Autodesk Fusion 360 part; units mm, degrees
(part 15 of 20)
  line L330 (29.8938, -739.4997) -> (29.2799, -739.4997)
  line L331 (20.1598, -739.4999) -> (19.5459, -739.4999)
  line L332 (19.5459, -739.4999) -> (19.5458, -735.5879)
  spline S948 degree 3 poles (19.5458, -735.5879) (19.4621, -735.6608) (19.2807, -735.8186) (19.0751, -735.9436) (18.9643, -736.0109) knots 0 0 0 0 0.033221 0.072019 0.072019 0.072019 0.072019
  spline S949 degree 3 poles (18.9643, -736.0109) (18.8518, -736.0753) (18.6431, -736.1948) (18.4206, -736.286) (18.318, -736.3281) knots 0 0 0 0 0.03884 0.072064 0.072064 0.072064 0.072064
  line L333 (18.318, -736.3281) -> (18.318, -735.7346)
  spline S950 degree 3 poles (18.318, -735.7346) (18.4826, -735.6511) (18.804, -735.488) (19.0825, -735.2595) (19.2184, -735.148) knots 0 0 0 0 0.05519 0.10775 0.10775 0.10775 0.10775
  spline S951 degree 3 poles (19.2184, -735.148) (19.3344, -735.0399) (19.5471, -734.8418) (19.6962, -734.5927) (19.7641, -734.4795) knots 0 0 0 0 0.047275 0.086674 0.086674 0.086674 0.086674
  line L334 (19.7641, -734.4795) -> (20.1597, -734.4795)
  line L335 (20.1597, -734.4795) -> (20.1598, -739.4999)
  line L336 (28.5502, -789.465) -> (28.5499, -785.8429)
  line L337 (28.5499, -785.8429) -> (29.0991, -785.8429)
  line L338 (29.0991, -785.8429) -> (29.0991, -786.3511)
  spline S952 degree 3 poles (29.0991, -786.3511) (29.161, -786.2665) (29.2859, -786.096) (29.4633, -785.981) (29.5527, -785.923) knots 0 0 0 0 0.031158 0.062835 0.062835 0.062835 0.062835
  spline S953 degree 3 poles (29.5527, -785.923) (29.6519, -785.8758) (29.8557, -785.7786) (30.0814, -785.767) (30.1973, -785.761) knots 0 0 0 0 0.032617 0.067048 0.067048 0.067048 0.067048
  spline S954 degree 3 poles (30.1973, -785.761) (30.3218, -785.7657) (30.5542, -785.7745) (30.7612, -785.8794) (30.8572, -785.928) knots 0 0 0 0 0.036859 0.068796 0.068796 0.068796 0.068796
  spline S955 degree 3 poles (30.8572, -785.928) (30.9369, -785.9898) (31.0979, -786.1144) (31.1794, -786.301) (31.2205, -786.3953) knots 0 0 0 0 0.029725 0.060035 0.060035 0.060035 0.060035
  spline S956 degree 3 poles (31.2205, -786.3953) (31.3707, -786.2103) (31.6618, -785.8517) (32.1182, -785.7905) (32.3392, -785.7608) knots 0 0 0 0 0.068625 0.133023 0.133023 0.133023 0.133023
  spline S957 degree 3 poles (32.3392, -785.7608) (32.5042, -785.7692) (32.8121, -785.7849) (33.0552, -785.9723) (33.168, -786.0592) knots 0 0 0 0 0.048244 0.08997 0.08997 0.08997 0.08997
  spline S958 degree 3 poles (33.168, -786.0592) (33.2523, -786.1815) (33.4417, -786.4564) (33.4522, -786.792) (33.4579, -786.9783) knots 0 0 0 0 0.043695 0.098195 0.098195 0.098195 0.098195
  line L339 (33.4579, -786.9783) -> (33.4581, -789.4647)
  line L340 (33.4581, -789.4647) -> (32.8476, -789.4647)
  line L341 (32.8476, -789.4647) -> (32.8475, -787.183)
  spline S959 degree 3 poles (32.8475, -787.183) (32.8474, -787.0768) (32.8474, -786.8975) (32.805, -786.7235) (32.7877, -786.6526) knots 0 0 0 0 0.031711 0.053535 0.053535 0.053535 0.053535
  spline S960 degree 3 poles (32.7877, -786.6526) (32.7633, -786.601) (32.7134, -786.4956) (32.6192, -786.4268) (32.5711, -786.3918) knots 0 0 0 0 0.016863 0.034394 0.034394 0.034394 0.034394
  spline S961 degree 3 poles (32.5711, -786.3918) (32.5154, -786.3629) (32.4, -786.3032) (32.27, -786.2964) (32.2028, -786.2929) knots 0 0 0 0 0.018597 0.038532 0.038532 0.038532 0.038532
  spline S962 degree 3 poles (32.2028, -786.2929) (32.0816, -786.3027) (31.8437, -786.3219) (31.6591, -786.4729) (31.5684, -786.547) knots 0 0 0 0 0.035532 0.069798 0.069798 0.069798 0.069798
  spline S963 degree 3 poles (31.5684, -786.547) (31.4951, -786.6537) (31.328, -786.8969) (31.3204, -787.1938) (31.3161, -787.3605) knots 0 0 0 0 0.038079 0.086792 0.086792 0.086792 0.086792
  line L342 (31.3161, -787.3605) -> (31.3162, -789.4648)
  line L343 (31.3162, -789.4648) -> (30.7023, -789.4649)
  line L344 (30.7023, -789.4649) -> (30.7022, -787.1115)
  spline S964 degree 3 poles (30.7022, -787.1115) (30.6997, -786.9895) (30.6954, -786.7727) (30.5956, -786.5813) (30.552, -786.4976) knots 0 0 0 0 0.036008 0.063954 0.063954 0.063954 0.063954
  spline S965 degree 3 poles (30.552, -786.4976) (30.4898, -786.4381) (30.3536, -786.3077) (30.1639, -786.2982) (30.0609, -786.293) knots 0 0 0 0 0.025037 0.054812 0.054812 0.054812 0.054812
  spline S966 degree 3 poles (30.0609, -786.293) (29.9761, -786.2987) (29.8067, -786.3101) (29.6567, -786.3897) (29.5817, -786.4295) knots 0 0 0 0 0.025172 0.050327 0.050327 0.050327 0.050327
  spline S967 degree 3 poles (29.5817, -786.4295) (29.5131, -786.4812) (29.3728, -786.5868) (29.3, -786.7468) (29.2628, -786.8286) knots 0 0 0 0 0.025339 0.051812 0.051812 0.051812 0.051812
  spline S968 degree 3 poles (29.2628, -786.8286) (29.2341, -786.9349) (29.1673, -787.1824) (29.1652, -787.4392) (29.164, -787.5857) knots 0 0 0 0 0.032907 0.076633 0.076633 0.076633 0.076633
  line L345 (29.164, -787.5857) -> (29.1641, -789.465)
  line L346 (29.1641, -789.465) -> (28.5502, -789.465)
  line L347 (27.416, -838.1729) -> (28.0197, -838.2513)
  spline S969 degree 3 poles (28.0197, -838.2513) (27.9771, -838.4452) (27.8953, -838.817) (27.6369, -839.0953) (27.5133, -839.2285) knots 0 0 0 0 0.058356 0.111856 0.111856 0.111856 0.111856
  spline S970 degree 3 poles (27.5133, -839.2285) (27.3672, -839.3314) (27.0671, -839.5429) (26.7004, -839.5684) (26.5123, -839.5815) knots 0 0 0 0 0.052559 0.107965 0.107965 0.107965 0.107965
  spline S971 degree 3 poles (26.5123, -839.5815) (26.2792, -839.564) (25.8276, -839.5301) (25.4834, -839.2373) (25.3168, -839.0956) knots 0 0 0 0 0.068154 0.132052 0.132052 0.132052 0.132052
  spline S972 degree 3 poles (25.3168, -839.0956) (25.1853, -838.9048) (24.8974, -838.4874) (24.8763, -837.9786) (24.8649, -837.7023) knots 0 0 0 0 0.068157 0.149141 0.149141 0.149141 0.149141
  spline S973 degree 3 poles (24.8649, -837.7023) (24.8712, -837.5171) (24.8832, -837.1646) (25.0026, -836.833) (25.0592, -836.6757) knots 0 0 0 0 0.055211 0.105055 0.105055 0.105055 0.105055
  spline S974 degree 3 poles (25.0592, -836.6757) (25.1314, -836.5388) (25.2736, -836.2692) (25.5265, -836.0993) (25.651, -836.0157) knots 0 0 0 0 0.04564 0.089884 0.089884 0.089884 0.089884
  spline S975 degree 3 poles (25.651, -836.0157) (25.7869, -835.9516) (26.0608, -835.8223) (26.3632, -835.8046) (26.5156, -835.7957) knots 0 0 0 0 0.044643 0.089955 0.089955 0.089955 0.089955
  spline S976 degree 3 poles (26.5156, -835.7957) (26.6993, -835.8051) (27.0472, -835.8228) (27.3418, -836.0071) (27.4808, -836.0941) knots 0 0 0 0 0.054149 0.102527 0.102527 0.102527 0.102527
  spline S977 degree 3 poles (27.4808, -836.0941) (27.5953, -836.2076) (27.8343, -836.4446) (27.9181, -836.7714) (27.9617, -836.9416) knots 0 0 0 0 0.047449 0.099081 0.099081 0.099081 0.099081
  line L348 (27.9617, -836.9416) -> (27.3648, -837.0337)
  spline S978 degree 3 poles (27.3648, -837.0337) (27.334, -836.9224) (27.2765, -836.7149) (27.1306, -836.5575) (27.063, -836.4846) knots 0 0 0 0 0.034086 0.063475 0.063475 0.063475 0.063475
  spline S979 degree 3 poles (27.063, -836.4846) (26.986, -836.4309) (26.8287, -836.3212) (26.6372, -836.3075) (26.5394, -836.3005) knots 0 0 0 0 0.027619 0.056426 0.056426 0.056426 0.056426
  spline S980 degree 3 poles (26.5394, -836.3005) (26.3928, -836.3135) (26.1037, -836.3393) (25.8907, -836.5361) (25.7857, -836.6331) knots 0 0 0 0 0.04285 0.084486 0.084486 0.084486 0.084486
  spline S981 degree 3 poles (25.7857, -836.6331) (25.7015, -836.7726) (25.5077, -837.0941) (25.5001, -837.4716) (25.4958, -837.6852) knots 0 0 0 0 0.048123 0.11083 0.11083 0.11083 0.11083
  spline S982 degree 3 poles (25.4958, -837.6852) (25.4994, -837.901) (25.5057, -838.2797) (25.6944, -838.6057) (25.7755, -838.7459) knots 0 0 0 0 0.063398 0.111295 0.111295 0.111295 0.111295
  spline S983 degree 3 poles (25.7755, -838.7459) (25.8767, -838.8424) (26.0813, -839.0376) (26.363, -839.0636) (26.5054, -839.0768) knots 0 0 0 0 0.040675 0.082263 0.082263 0.082263 0.082263
  spline S984 degree 3 poles (26.5054, -839.0768) (26.6198, -839.0685) (26.8427, -839.0525) (27.0219, -838.9197) (27.1091, -838.855) knots 0 0 0 0 0.033628 0.065508 0.065508 0.065508 0.065508
  spline S985 degree 3 poles (27.1091, -838.855) (27.1832, -838.7651) (27.3466, -838.5664) (27.3915, -838.312) (27.416, -838.1729) knots 0 0 0 0 0.034396 0.07593 0.07593 0.07593 0.07593
  spline S986 degree 3 poles (19.0565, -837.034) (19.0601, -836.7657) (19.0666, -836.2825) (19.1859, -835.8147) (19.2389, -835.6067) knots 0 0 0 0 0.080152 0.144341 0.144341 0.144341 0.144341
  spline S987 degree 3 poles (19.2389, -835.6067) (19.3036, -835.4398) (19.4261, -835.1233) (19.6672, -834.8853) (19.7812, -834.7728) knots 0 0 0 0 0.052977 0.10048 0.10048 0.10048 0.10048
  spline S988 degree 3 poles (19.7812, -834.7728) (19.9126, -834.6872) (20.1874, -834.5083) (20.5155, -834.4893) (20.6867, -834.4794) knots 0 0 0 0 0.046203 0.096661 0.096661 0.096661 0.096661
  spline S989 degree 3 poles (20.6867, -834.4794) (20.8145, -834.485) (21.06, -834.4957) (21.2849, -834.5942) (21.3927, -834.6414) knots 0 0 0 0 0.037989 0.072993 0.072993 0.072993 0.072993
  spline S990 degree 3 poles (21.3927, -834.6414) (21.49, -834.7021) (21.6873, -834.8253) (21.8245, -835.0133) (21.8941, -835.1086) knots 0 0 0 0 0.034048 0.069103 0.069103 0.069103 0.069103
  spline S991 degree 3 poles (21.8941, -835.1086) (21.9574, -835.2196) (22.0914, -835.4545) (22.1655, -835.7148) (22.2045, -835.8521) knots 0 0 0 0 0.038176 0.080832 0.080832 0.080832 0.080832
  spline S992 degree 3 poles (22.2045, -835.8521) (22.2372, -836.0232) (22.3118, -836.4133) (22.3152, -836.8108) (22.3171, -837.0339) knots 0 0 0 0 0.052146 0.118926 0.118926 0.118926 0.118926
  spline S993 degree 3 poles (22.3171, -837.0339) (22.3135, -837.3005) (22.3069, -837.7813) (22.1889, -838.247) (22.1364, -838.4545) knots 0 0 0 0 0.079639 0.143634 0.143634 0.143634 0.143634
  spline S994 degree 3 poles (22.1364, -838.4545) (22.0722, -838.6214) (21.9504, -838.9384) (21.7097, -839.1771) (21.5958, -839.2901) knots 0 0 0 0 0.052961 0.100531 0.100531 0.100531 0.100531
  spline S995 degree 3 poles (21.5958, -839.2901) (21.4642, -839.3761) (21.1885, -839.5562) (20.8591, -839.5752) (20.6869, -839.5851) knots 0 0 0 0 0.046339 0.097057 0.097057 0.097057 0.097057
  spline S996 degree 3 poles (20.6869, -839.5851) (20.4607, -839.5658) (20.0194, -839.5282) (19.7046, -839.2179) (19.5511, -839.0668) knots 0 0 0 0 0.065835 0.128409 0.128409 0.128409 0.128409
  spline S997 degree 3 poles (19.5511, -839.0668) (19.4077, -838.7987) (19.0701, -838.1677) (19.0615, -837.448) (19.0565, -837.034) knots 0 0 0 0 0.090022 0.211899 0.211899 0.211899 0.211899
  line L349 (5, 0) -> (5, -3)
  line L350 (5, -3) -> (0, -3)
  line L351 (0, -3) -> (0, -36.5)
  line L352 (0, -36.5) -> (17.5, -36.5)
  line L353 (17.5, -36.5) -> (17.5, -37.5)
  line L354 (17.5, -37.5) -> (0, -37.5)
  line L355 (0, -37.5) -> (0, -46.5)
  line L356 (0, -46.5) -> (17.5, -46.5)
  line L357 (17.5, -46.5) -> (17.5, -47.5)
  line L358 (17.5, -47.5) -> (0, -47.5)
  line L359 (0, -47.5) -> (0, -56.5)
  line L360 (0, -56.5) -> (17.5, -56.5)
  line L361 (17.5, -56.5) -> (17.5, -57.5)
  line L362 (17.5, -57.5) -> (0, -57.5)
  line L363 (0, -57.5) -> (0, -66.5)
  line L364 (0, -66.5) -> (17.5, -66.5)
  line L365 (17.5, -66.5) -> (17.5, -67.5)
  line L366 (17.5, -67.5) -> (0, -67.5)
  line L367 (0, -67.5) -> (0, -76.5)
  line L368 (0, -76.5) -> (17.5, -76.5)
  line L369 (17.5, -76.5) -> (17.5, -77.5)
  line L370 (17.5, -77.5) -> (0, -77.5)
  line L371 (0, -77.5) -> (0, -86.5)
  line L372 (0, -86.5) -> (17.5, -86.5)
  line L373 (17.5, -86.5) -> (17.5, -87.5)
  line L374 (17.5, -87.5) -> (0, -87.5)
  line L375 (0, -87.5) -> (0, -96.5)
  line L376 (0, -96.5) -> (17.5, -96.5)
  line L377 (17.5, -96.5) -> (17.5, -97.5)
  line L378 (17.5, -97.5) -> (0, -97.5)
  line L379 (0, -97.5) -> (0, -106.5)
  line L380 (0, -106.5) -> (17.5, -106.5)
  line L381 (17.5, -106.5) -> (17.5, -107.5)
  line L382 (17.5, -107.5) -> (0, -107.5)
  line L383 (0, -107.5) -> (0, -116.5)
  line L384 (0, -116.5) -> (17.5, -116.5)
  line L385 (17.5, -116.5) -> (17.5, -117.5)
  line L386 (17.5, -117.5) -> (0, -117.5)
  line L387 (0, -117.5) -> (0, -126.5)
  line L388 (0, -126.5) -> (17.5, -126.5)
  line L389 (17.5, -126.5) -> (17.5, -127.5)
  line L390 (17.5, -127.5) -> (0, -127.5)
  line L391 (0, -127.5) -> (0, -136.5)
  line L392 (0, -136.5) -> (17.5, -136.5)
  line L393 (17.5, -136.5) -> (17.5, -137.5)
  line L394 (17.5, -137.5) -> (0, -137.5)
  line L395 (0, -137.5) -> (0, -146.5)
  line L396 (0, -146.5) -> (17.5, -146.5)
  line L397 (17.5, -146.5) -> (17.5, -147.5)
  line L398 (17.5, -147.5) -> (0, -147.5)
  line L399 (0, -147.5) -> (0, -156.5)
  line L400 (0, -156.5) -> (17.5, -156.5)
  line L401 (17.5, -156.5) -> (17.5, -157.5)
  line L402 (17.5, -157.5) -> (0, -157.5)
  line L403 (0, -157.5) -> (0, -166.5)
  line L404 (0, -166.5) -> (17.5, -166.5)
  line L405 (17.5, -166.5) -> (17.5, -167.5)
  line L406 (17.5, -167.5) -> (0, -167.5)
  line L407 (0, -167.5) -> (0, -176.5)
  line L408 (0, -176.5) -> (17.5, -176.5)
  line L409 (17.5, -176.5) -> (17.5, -177.5)
  line L410 (17.5, -177.5) -> (0, -177.5)
  line L411 (0, -177.5) -> (0, -186.5)
  line L412 (0, -186.5) -> (17.5, -186.5)
  line L413 (17.5, -186.5) -> (17.5, -187.5)
  line L414 (17.5, -187.5) -> (0, -187.5)
  line L415 (0, -187.5) -> (0, -196.5)
  line L416 (0, -196.5) -> (17.5, -196.5)
  line L417 (17.5, -196.5) -> (17.5, -197.5)
  line L418 (17.5, -197.5) -> (0, -197.5)
  line L419 (0, -197.5) -> (0, -206.5)
  line L420 (0, -206.5) -> (17.5, -206.5)
  line L421 (17.5, -206.5) -> (17.5, -207.5)
  line L422 (17.5, -207.5) -> (0, -207.5)
  line L423 (0, -207.5) -> (0, -216.5)
  line L424 (0, -216.5) -> (17.5, -216.5)
  line L425 (17.5, -216.5) -> (17.5, -217.5)
  line L426 (17.5, -217.5) -> (0, -217.5)
  line L427 (0, -217.5) -> (0, -226.5)
  line L428 (0, -226.5) -> (17.5, -226.5)
  line L429 (17.5, -226.5) -> (17.5, -227.5)
  line L430 (17.5, -227.5) -> (0, -227.5)
  line L431 (0, -227.5) -> (0, -236.5)
  line L432 (0, -236.5) -> (17.5, -236.5)
  line L433 (17.5, -236.5) -> (17.5, -237.5)
  line L434 (17.5, -237.5) -> (0, -237.5)
  line L435 (0, -237.5) -> (0, -246.5)
  line L436 (0, -246.5) -> (17.5, -246.5)
  line L437 (17.5, -246.5) -> (17.5, -247.5)
  line L438 (17.5, -247.5) -> (0, -247.5)
  line L439 (0, -247.5) -> (0, -256.5)
  line L440 (0, -256.5) -> (17.5, -256.5)
  line L441 (17.5, -256.5) -> (17.5, -257.5)
  line L442 (17.5, -257.5) -> (0, -257.5)
  line L443 (0, -257.5) -> (0, -266.5)
  line L444 (0, -266.5) -> (17.5, -266.5)
  line L445 (17.5, -266.5) -> (17.5, -267.5)
  line L446 (17.5, -267.5) -> (0, -267.5)
  line L447 (0, -267.5) -> (0, -276.5)
  line L448 (0, -276.5) -> (17.5, -276.5)
  line L449 (17.5, -276.5) -> (17.5, -277.5)
  line L450 (17.5, -277.5) -> (0, -277.5)
  line L451 (0, -277.5) -> (0, -286.5)
  line L452 (0, -286.5) -> (17.5, -286.5)
  line L453 (17.5, -286.5) -> (17.5, -287.5)
  line L454 (17.5, -287.5) -> (0, -287.5)
  line L455 (0, -287.5) -> (0, -296.5)
  line L456 (0, -296.5) -> (17.5, -296.5)
  line L457 (17.5, -296.5) -> (17.5, -297.5)
  line L458 (17.5, -297.5) -> (0, -297.5)
  line L459 (0, -297.5) -> (0, -306.5)
  line L460 (0, -306.5) -> (17.5, -306.5)
  line L461 (17.5, -306.5) -> (17.5, -307.5)
  line L462 (17.5, -307.5) -> (0, -307.5)
  line L463 (0, -307.5) -> (0, -316.5)
  line L464 (0, -316.5) -> (17.5, -316.5)
  line L465 (17.5, -316.5) -> (17.5, -317.5)
  line L466 (17.5, -317.5) -> (0, -317.5)
  line L467 (0, -317.5) -> (0, -326.5)
  line L468 (0, -326.5) -> (17.5, -326.5)
  line L469 (17.5, -326.5) -> (17.5, -327.5)
  line L470 (17.5, -327.5) -> (0, -327.5)
  line L471 (0, -327.5) -> (0, -336.5)
  line L472 (0, -336.5) -> (17.5, -336.5)
  line L473 (17.5, -336.5) -> (17.5, -337.5)
  line L474 (17.5, -337.5) -> (0, -337.5)
  line L475 (0, -337.5) -> (0, -346.5)
  line L476 (0, -346.5) -> (17.5, -346.5)
  line L477 (17.5, -346.5) -> (17.5, -347.5)
  line L478 (17.5, -347.5) -> (0, -347.5)
  line L479 (0, -347.5) -> (0, -356.5)
  line L480 (0, -356.5) -> (17.5, -356.5)
  line L481 (17.5, -356.5) -> (17.5, -357.5)
  line L482 (17.5, -357.5) -> (0, -357.5)
  line L483 (0, -357.5) -> (0, -366.5)
  line L484 (0, -366.5) -> (17.5, -366.5)
  line L485 (17.5, -366.5) -> (17.5, -367.5)
  line L486 (17.5, -367.5) -> (0, -367.5)
  line L487 (0, -367.5) -> (0, -376.5)
  line L488 (0, -376.5) -> (17.5, -376.5)
  line L489 (17.5, -376.5) -> (17.5, -377.5)
  line L490 (17.5, -377.5) -> (0, -377.5)
  line L491 (0, -377.5) -> (0, -386.5)
  line L492 (0, -386.5) -> (17.5, -386.5)
  line L493 (17.5, -386.5) -> (17.5, -387.5)
  line L494 (17.5, -387.5) -> (0, -387.5)
  line L495 (0, -387.5) -> (0, -396.5)
  line L496 (0, -396.5) -> (17.5, -396.5)
  line L497 (17.5, -396.5) -> (17.5, -397.5)
  line L498 (17.5, -397.5) -> (0, -397.5)
  line L499 (0, -397.5) -> (0, -406.5)
  line L500 (0, -406.5) -> (17.5, -406.5)
  line L501 (17.5, -406.5) -> (17.5, -407.5)
  line L502 (17.5, -407.5) -> (0, -407.5)
  line L503 (0, -407.5) -> (0, -416.5)
  line L504 (0, -416.5) -> (17.5, -416.5)
  line L505 (17.5, -416.5) -> (17.5, -417.5)
  line L506 (17.5, -417.5) -> (0, -417.5)
  line L507 (0, -417.5) -> (0, -426.5)
  line L508 (0, -426.5) -> (17.5, -426.5)
  line L509 (17.5, -426.5) -> (17.5, -427.5)
  line L510 (17.5, -427.5) -> (0, -427.5)
  line L511 (0, -427.5) -> (0, -436.5)
  line L512 (0, -436.5) -> (17.5, -436.5)
  line L513 (17.5, -436.5) -> (17.5, -437.5)
  line L514 (17.5, -437.5) -> (0, -437.5)
  line L515 (0, -437.5) -> (0, -446.5)
  line L516 (0, -446.5) -> (17.5, -446.5)
  line L517 (17.5, -446.5) -> (17.5, -447.5)
  line L518 (17.5, -447.5) -> (0, -447.5)
  line L519 (0, -447.5) -> (0, -456.5)
  line L520 (0, -456.5) -> (17.5, -456.5)
  line L521 (17.5, -456.5) -> (17.5, -457.5)
  line L522 (17.5, -457.5) -> (0, -457.5)
  line L523 (0, -457.5) -> (0, -466.5)
  line L524 (0, -466.5) -> (17.5, -466.5)
  line L525 (17.5, -466.5) -> (17.5, -467.5)
  line L526 (17.5, -467.5) -> (0, -467.5)
  line L527 (0, -467.5) -> (0, -476.5)
  line L528 (0, -476.5) -> (17.5, -476.5)
  line L529 (17.5, -476.5) -> (17.5, -477.5)
  line L530 (17.5, -477.5) -> (0, -477.5)
  line L531 (0, -477.5) -> (0, -486.5)
  line L532 (0, -486.5) -> (17.5, -486.5)
  line L533 (17.5, -486.5) -> (17.5, -487.5)
  line L534 (17.5, -487.5) -> (0, -487.5)
  line L535 (0, -487.5) -> (0, -496.5)
  line L536 (0, -496.5) -> (17.5, -496.5)
  line L537 (17.5, -496.5) -> (17.5, -497.5)
  line L538 (17.5, -497.5) -> (0, -497.5)
  line L539 (0, -497.5) -> (0, -506.5)
  line L540 (0, -506.5) -> (17.5, -506.5)
  line L541 (17.5, -506.5) -> (17.5, -507.5)
  line L542 (17.5, -507.5) -> (0, -507.5)
  line L543 (0, -507.5) -> (0, -516.5)
  line L544 (0, -516.5) -> (17.5, -516.5)
  line L545 (17.5, -516.5) -> (17.5, -517.5)
  line L546 (17.5, -517.5) -> (0, -517.5)
  line L547 (0, -517.5) -> (0, -526.5)
  line L548 (0, -526.5) -> (17.5, -526.5)
  line L549 (17.5, -526.5) -> (17.5, -527.5)
  line L550 (17.5, -527.5) -> (0, -527.5)
  line L551 (0, -527.5) -> (0, -536.5)
  line L552 (0, -536.5) -> (17.5, -536.5)
  line L553 (17.5, -536.5) -> (17.5, -537.5)
  line L554 (17.5, -537.5) -> (0, -537.5)
  line L555 (0, -537.5) -> (0, -546.5)
  line L556 (0, -546.5) -> (17.5, -546.5)
  line L557 (17.5, -546.5) -> (17.5, -547.5)
  line L558 (17.5, -547.5) -> (0, -547.5)
  line L559 (0, -547.5) -> (0, -556.5)
  line L560 (0, -556.5) -> (17.5, -556.5)
  line L561 (17.5, -556.5) -> (17.5, -557.5)
  line L562 (17.5, -557.5) -> (0, -557.5)
  line L563 (0, -557.5) -> (0, -566.5)
  line L564 (0, -566.5) -> (17.5, -566.5)
  line L565 (17.5, -566.5) -> (17.5, -567.5)
  line L566 (17.5, -567.5) -> (0, -567.5)
  line L567 (0, -567.5) -> (0, -576.5)
  line L568 (0, -576.5) -> (17.5, -576.5)
  line L569 (17.5, -576.5) -> (17.5, -577.5)
  line L570 (17.5, -577.5) -> (0, -577.5)
  line L571 (0, -577.5) -> (0, -586.5)
  line L572 (0, -586.5) -> (17.5, -586.5)
  line L573 (17.5, -586.5) -> (17.5, -587.5)
  line L574 (17.5, -587.5) -> (0, -587.5)
  line L575 (0, -587.5) -> (0, -596.5)
  line L576 (0, -596.5) -> (17.5, -596.5)
  line L577 (17.5, -596.5) -> (17.5, -597.5)
  line L578 (17.5, -597.5) -> (0, -597.5)
  line L579 (0, -597.5) -> (0, -606.5)
  line L580 (0, -606.5) -> (17.5, -606.5)
  line L581 (17.5, -606.5) -> (17.5, -607.5)
  line L582 (17.5, -607.5) -> (0, -607.5)
  line L583 (0, -607.5) -> (0, -616.5)
  line L584 (0, -616.5) -> (17.5, -616.5)
  line L585 (17.5, -616.5) -> (17.5, -617.5)
  line L586 (17.5, -617.5) -> (0, -617.5)
  line L587 (0, -617.5) -> (0, -626.5)
  line L588 (0, -626.5) -> (17.5, -626.5)
  line L589 (17.5, -626.5) -> (17.5, -627.5)
  line L590 (17.5, -627.5) -> (0, -627.5)
  line L591 (0, -627.5) -> (0, -636.5)
  line L592 (0, -636.5) -> (17.5, -636.5)
  line L593 (17.5, -636.5) -> (17.5, -637.5)
  line L594 (17.5, -637.5) -> (0, -637.5)
  line L595 (0, -637.5) -> (0, -646.5)
  line L596 (0, -646.5) -> (17.5, -646.5)
  line L597 (17.5, -646.5) -> (17.5, -647.5)
  line L598 (17.5, -647.5) -> (0, -647.5)
  line L599 (0, -647.5) -> (0, -656.5)
  line L600 (0, -656.5) -> (17.5, -656.5)
  line L601 (17.5, -656.5) -> (17.5, -657.5)
  line L602 (17.5, -657.5) -> (0, -657.5)
  line L603 (0, -657.5) -> (0, -666.5)
  line L604 (0, -666.5) -> (17.5, -666.5)
  line L605 (17.5, -666.5) -> (17.5, -667.5)
  line L606 (17.5, -667.5) -> (0, -667.5)
  line L607 (0, -667.5) -> (0, -676.5)
  line L608 (0, -676.5) -> (17.5, -676.5)
  line L609 (17.5, -676.5) -> (17.5, -677.5)
  line L610 (17.5, -677.5) -> (0, -677.5)
  line L611 (0, -677.5) -> (0, -686.5)
  line L612 (0, -686.5) -> (17.5, -686.5)
  line L613 (17.5, -686.5) -> (17.5, -687.5)
  line L614 (17.5, -687.5) -> (0, -687.5)
  line L615 (0, -687.5) -> (0, -696.5)
  line L616 (0, -696.5) -> (17.5, -696.5)
  line L617 (17.5, -696.5) -> (17.5, -697.5)
  line L618 (17.5, -697.5) -> (0, -697.5)
  line L619 (0, -697.5) -> (0, -706.5)
  line L620 (0, -706.5) -> (17.5, -706.5)
  line L621 (17.5, -706.5) -> (17.5, -707.5)
  line L622 (17.5, -707.5) -> (0, -707.5)
  line L623 (0, -707.5) -> (0, -716.5)
  line L624 (0, -716.5) -> (17.5, -716.5)
  line L625 (17.5, -716.5) -> (17.5, -717.5)
  line L626 (17.5, -717.5) -> (0, -717.5)
  line L627 (0, -717.5) -> (0, -726.5)
  line L628 (0, -726.5) -> (17.5, -726.5)
  line L629 (17.5, -726.5) -> (17.5, -727.5)
  line L630 (17.5, -727.5) -> (0, -727.5)
  line L631 (0, -727.5) -> (0, -736.5)
  line L632 (0, -736.5) -> (17.5, -736.5)
  line L633 (17.5, -736.5) -> (17.5, -737.5)
  line L634 (17.5, -737.5) -> (0, -737.5)
  line L635 (0, -737.5) -> (0, -746.5)
  line L636 (0, -746.5) -> (17.5, -746.5)
  line L637 (17.5, -746.5) -> (17.5, -747.5)
  line L638 (17.5, -747.5) -> (0, -747.5)
  line L639 (0, -747.5) -> (0, -756.5)
  line L640 (0, -756.5) -> (17.5, -756.5)
  line L641 (17.5, -756.5) -> (17.5, -757.5)
  line L642 (17.5, -757.5) -> (0, -757.5)
  line L643 (0, -757.5) -> (0, -766.5)
  line L644 (0, -766.5) -> (17.5, -766.5)
  line L645 (17.5, -766.5) -> (17.5, -767.5)
  line L646 (17.5, -767.5) -> (0, -767.5)
  line L647 (0, -767.5) -> (0, -776.5)
  line L648 (0, -776.5) -> (17.5, -776.5)
  line L649 (17.5, -776.5) -> (17.5, -777.5)
  line L650 (17.5, -777.5) -> (0, -777.5)
  line L651 (0, -777.5) -> (0, -786.5)
  line L652 (0, -786.5) -> (17.5, -786.5)
  line L653 (17.5, -786.5) -> (17.5, -787.5)
  line L654 (17.5, -787.5) -> (0, -787.5)
  line L655 (0, -787.5) -> (0, -796.5)
  line L656 (0, -796.5) -> (17.5, -796.5)
  line L657 (17.5, -796.5) -> (17.5, -797.5)
  line L658 (17.5, -797.5) -> (0, -797.5)
  line L659 (0, -797.5) -> (0, -806.5)
  line L660 (0, -806.5) -> (17.5, -806.5)
  line L661 (17.5, -806.5) -> (17.5, -807.5)
  line L662 (17.5, -807.5) -> (0, -807.5)
  line L663 (0, -807.5) -> (0, -816.5)
  line L664 (0, -816.5) -> (17.5, -816.5)
  line L665 (17.5, -816.5) -> (17.5, -817.5)
  line L666 (17.5, -817.5) -> (0, -817.5)
  line L667 (0, -817.5) -> (0, -826.5)
  line L668 (0, -826.5) -> (17.5, -826.5)
  line L669 (17.5, -826.5) -> (17.5, -827.5)
  line L670 (17.5, -827.5) -> (0, -827.5)
  line L671 (0, -827.5) -> (0, -836.5)
  line L672 (0, -836.5) -> (17.5, -836.5)
  line L673 (17.5, -836.5) -> (17.5, -837.5)
  line L674 (17.5, -837.5) -> (0, -837.5)
  line L675 (0, -837.5) -> (0, -870.7)
  line L676 (0, -870.7) -> (5, -870.7)
  line L677 (5, -870.7) -> (5, -874)
  line L678 (5, -874) -> (35, -874)
  line L679 (35, -874) -> (35, -870.7)
  line L680 (35, -870.7) -> (40, -870.7)
  line L681 (40, -870.7) -> (40, -3)
  line L682 (40, -3) -> (35, -3)
  line L683 (35, -3) -> (35, 0)
  line L684 (35, 0) -> (5, 0)
  line L685 (5, 0) -> (5, 10)
  line L686 (5, 10) -> (35, 10)
  line L687 (35, 10) -> (35, 0)
  line L688 (27.5, 3) -> (12.5, 3)
  line L689 (12.5, 3) -> (12.5, 0)
  line L690 (12.5, 0) -> (27.5, 0)
  line L691 (27.5, 0) -> (27.5, 3)
  line L692 (27.5, 3) -> (12.5, 0) construction
  line L693 (12.5, 3) -> (27.5, 0) construction
  line L694 (5, -874) -> (5, -884)
  line L695 (5, -884) -> (35, -884)
  line L696 (35, -884) -> (35, -874)
  point P0 (20, 1.5)
  dimension "d265" = 10
  dimension "d266" = 3
  dimension "d267" = 15
  dimension "d268" = 15
  dimension "d269" = 7
  constraint coincident L349.start L684.end
  constraint perpendicular L684 L685
  constraint perpendicular L685 L686
  constraint coincident L683.end L684.start
  constraint perpendicular L684 L687
  constraint horizontal L688
  constraint perpendicular L688 L689
  constraint parallel L688 L690
  constraint parallel L689 L691
  constraint coincident L692 P0
  constraint coincident L693 P0
  constraint coincident L677.end L678.start
  constraint perpendicular L678 L694
  constraint perpendicular L677 L695
  constraint coincident L678.end L679.start
  constraint perpendicular L678 L696
  measures "d265" distance of L349.start L685.end
  measures "d266" distance of L688.end L689.end
  measures "d267" distance of L688.start L688.end
  measures "d268" distance of L687 P0
  measures "d269" distance of L686 L688
extrude "Extruir9" add sketch "Boceto14" against normal blind 3 contours L684 L685 L686 L687 L688 L689 L691 | L678 L694 L695 L696
sketch "Boceto15" plane through (0, -1, 0) normal (0, -1, 0) x (1, 0, 0)
  line L0 (5, 10) -> (5, -3)
  line L1 (5, -3) -> (0, -3)
  line L2 (0, -3) -> (0, -36.5)
  line L3 (0, -36.5) -> (17.5, -36.5)
  line L4 (17.5, -36.5) -> (17.5, -37.5)
  line L5 (17.5, -37.5) -> (0, -37.5)
  line L6 (0, -37.5) -> (0, -46.5)
  line L7 (0, -46.5) -> (17.5, -46.5)
  line L8 (17.5, -46.5) -> (17.5, -47.5)
  line L9 (17.5, -47.5) -> (0, -47.5)
  line L10 (0, -47.5) -> (0, -56.5)
  line L11 (0, -56.5) -> (17.5, -56.5)
  line L12 (17.5, -56.5) -> (17.5, -57.5)
  line L13 (17.5, -57.5) -> (0, -57.5)
  line L14 (0, -57.5) -> (0, -66.5)
  line L15 (0, -66.5) -> (17.5, -66.5)
  line L16 (17.5, -66.5) -> (17.5, -67.5)
  line L17 (17.5, -67.5) -> (0, -67.5)
  line L18 (0, -67.5) -> (0, -76.5)
  line L19 (0, -76.5) -> (17.5, -76.5)
  line L20 (17.5, -76.5) -> (17.5, -77.5)
  line L21 (17.5, -77.5) -> (0, -77.5)
  line L22 (0, -77.5) -> (0, -86.5)
  line L23 (0, -86.5) -> (17.5, -86.5)
  line L24 (17.5, -86.5) -> (17.5, -87.5)
  line L25 (17.5, -87.5) -> (0, -87.5)
  line L26 (0, -87.5) -> (0, -96.5)
  line L27 (0, -96.5) -> (17.5, -96.5)
  line L28 (17.5, -96.5) -> (17.5, -97.5)
  line L29 (17.5, -97.5) -> (0, -97.5)
  line L30 (0, -97.5) -> (0, -106.5)
  line L31 (0, -106.5) -> (17.5, -106.5)
  line L32 (17.5, -106.5) -> (17.5, -107.5)
  line L33 (17.5, -107.5) -> (0, -107.5)
  line L34 (0, -107.5) -> (0, -116.5)
  line L35 (0, -116.5) -> (17.5, -116.5)
  line L36 (17.5, -116.5) -> (17.5, -117.5)
  line L37 (17.5, -117.5) -> (0, -117.5)
  line L38 (0, -117.5) -> (0, -126.5)
  line L39 (0, -126.5) -> (17.5, -126.5)
  line L40 (17.5, -126.5) -> (17.5, -127.5)
  line L41 (17.5, -127.5) -> (0, -127.5)
  line L42 (0, -127.5) -> (0, -136.5)
  line L43 (0, -136.5) -> (17.5, -136.5)
  line L44 (17.5, -136.5) -> (17.5, -137.5)
  line L45 (17.5, -137.5) -> (0, -137.5)
  line L46 (0, -137.5) -> (0, -146.5)
  line L47 (0, -146.5) -> (17.5, -146.5)
  line L48 (17.5, -146.5) -> (17.5, -147.5)
  line L49 (17.5, -147.5) -> (0, -147.5)
  line L50 (0, -147.5) -> (0, -156.5)
  line L51 (0, -156.5) -> (17.5, -156.5)
  line L52 (17.5, -156.5) -> (17.5, -157.5)
  line L53 (17.5, -157.5) -> (0, -157.5)
  line L54 (0, -157.5) -> (0, -166.5)
  line L55 (0, -166.5) -> (17.5, -166.5)
  line L56 (17.5, -166.5) -> (17.5, -167.5)
  line L57 (17.5, -167.5) -> (0, -167.5)
  line L58 (0, -167.5) -> (0, -176.5)
  line L59 (0, -176.5) -> (17.5, -176.5)
  line L60 (17.5, -176.5) -> (17.5, -177.5)
  line L61 (17.5, -177.5) -> (0, -177.5)
  line L62 (0, -177.5) -> (0, -186.5)
  line L63 (0, -186.5) -> (17.5, -186.5)
  line L64 (17.5, -186.5) -> (17.5, -187.5)
  line L65 (17.5, -187.5) -> (0, -187.5)
  line L66 (0, -187.5) -> (0, -196.5)
  line L67 (0, -196.5) -> (17.5, -196.5)
  line L68 (17.5, -196.5) -> (17.5, -197.5)
  line L69 (17.5, -197.5) -> (0, -197.5)
  line L70 (0, -197.5) -> (0, -206.5)
  line L71 (0, -206.5) -> (17.5, -206.5)
  line L72 (17.5, -206.5) -> (17.5, -207.5)
  line L73 (17.5, -207.5) -> (0, -207.5)
  line L74 (0, -207.5) -> (0, -216.5)
  line L75 (0, -216.5) -> (17.5, -216.5)
  line L76 (17.5, -216.5) -> (17.5, -217.5)
  line L77 (17.5, -217.5) -> (0, -217.5)
  line L78 (0, -217.5) -> (0, -226.5)
  line L79 (0, -226.5) -> (17.5, -226.5)
  line L80 (17.5, -226.5) -> (17.5, -227.5)
  line L81 (17.5, -227.5) -> (0, -227.5)
  line L82 (0, -227.5) -> (0, -236.5)
  line L83 (0, -236.5) -> (17.5, -236.5)
  line L84 (17.5, -236.5) -> (17.5, -237.5)
  line L85 (17.5, -237.5) -> (0, -237.5)
  line L86 (0, -237.5) -> (0, -246.5)
  line L87 (0, -246.5) -> (17.5, -246.5)
  line L88 (17.5, -246.5) -> (17.5, -247.5)
  line L89 (17.5, -247.5) -> (0, -247.5)
  line L90 (0, -247.5) -> (0, -256.5)
  line L91 (0, -256.5) -> (17.5, -256.5)
  line L92 (17.5, -256.5) -> (17.5, -257.5)
  line L93 (17.5, -257.5) -> (0, -257.5)
  line L94 (0, -257.5) -> (0, -266.5)
  line L95 (0, -266.5) -> (17.5, -266.5)
  line L96 (17.5, -266.5) -> (17.5, -267.5)
  line L97 (17.5, -267.5) -> (0, -267.5)
  line L98 (0, -267.5) -> (0, -276.5)
  line L99 (0, -276.5) -> (17.5, -276.5)
  line L100 (17.5, -276.5) -> (17.5, -277.5)
  line L101 (17.5, -277.5) -> (0, -277.5)
  line L102 (0, -277.5) -> (0, -286.5)
  line L103 (0, -286.5) -> (17.5, -286.5)
  line L104 (17.5, -286.5) -> (17.5, -287.5)
  line L105 (17.5, -287.5) -> (0, -287.5)
  line L106 (0, -287.5) -> (0, -296.5)
  line L107 (0, -296.5) -> (17.5, -296.5)
  line L108 (17.5, -296.5) -> (17.5, -297.5)
  line L109 (17.5, -297.5) -> (0, -297.5)
  line L110 (0, -297.5) -> (0, -306.5)
  line L111 (0, -306.5) -> (17.5, -306.5)
  line L112 (17.5, -306.5) -> (17.5, -307.5)
  line L113 (17.5, -307.5) -> (0, -307.5)
  line L114 (0, -307.5) -> (0, -316.5)
  line L115 (0, -316.5) -> (17.5, -316.5)
  line L116 (17.5, -316.5) -> (17.5, -317.5)
  line L117 (17.5, -317.5) -> (0, -317.5)
  line L118 (0, -317.5) -> (0, -326.5)
  line L119 (0, -326.5) -> (17.5, -326.5)
  line L120 (17.5, -326.5) -> (17.5, -327.5)
  line L121 (17.5, -327.5) -> (0, -327.5)
  line L122 (0, -327.5) -> (0, -336.5)
  line L123 (0, -336.5) -> (17.5, -336.5)
  line L124 (17.5, -336.5) -> (17.5, -337.5)
  line L125 (17.5, -337.5) -> (0, -337.5)
  line L126 (0, -337.5) -> (0, -346.5)
  line L127 (0, -346.5) -> (17.5, -346.5)
  line L128 (17.5, -346.5) -> (17.5, -347.5)
  line L129 (17.5, -347.5) -> (0, -347.5)
  line L130 (0, -347.5) -> (0, -356.5)
  line L131 (0, -356.5) -> (17.5, -356.5)
  line L132 (17.5, -356.5) -> (17.5, -357.5)
  line L133 (17.5, -357.5) -> (0, -357.5)
  line L134 (0, -357.5) -> (0, -366.5)
  line L135 (0, -366.5) -> (17.5, -366.5)
  line L136 (17.5, -366.5) -> (17.5, -367.5)
  line L137 (17.5, -367.5) -> (0, -367.5)
  line L138 (0, -367.5) -> (0, -376.5)
  line L139 (0, -376.5) -> (17.5, -376.5)
  line L140 (17.5, -376.5) -> (17.5, -377.5)
  line L141 (17.5, -377.5) -> (0, -377.5)
  line L142 (0, -377.5) -> (0, -386.5)
  line L143 (0, -386.5) -> (17.5, -386.5)
  line L144 (17.5, -386.5) -> (17.5, -387.5)
  line L145 (17.5, -387.5) -> (0, -387.5)
  line L146 (0, -387.5) -> (0, -396.5)
  line L147 (0, -396.5) -> (17.5, -396.5)
  line L148 (17.5, -396.5) -> (17.5, -397.5)
  line L149 (17.5, -397.5) -> (0, -397.5)
  line L150 (0, -397.5) -> (0, -406.5)
  line L151 (0, -406.5) -> (17.5, -406.5)
  line L152 (17.5, -406.5) -> (17.5, -407.5)
  line L153 (17.5, -407.5) -> (0, -407.5)
  line L154 (0, -407.5) -> (0, -416.5)
  line L155 (0, -416.5) -> (17.5, -416.5)
  line L156 (17.5, -416.5) -> (17.5, -417.5)
  line L157 (17.5, -417.5) -> (0, -417.5)
  line L158 (0, -417.5) -> (0, -426.5)
  line L159 (0, -426.5) -> (17.5, -426.5)
  line L160 (17.5, -426.5) -> (17.5, -427.5)
  line L161 (17.5, -427.5) -> (0, -427.5)
  line L162 (0, -427.5) -> (0, -436.5)
  line L163 (0, -436.5) -> (17.5, -436.5)
  line L164 (17.5, -436.5) -> (17.5, -437.5)
  line L165 (17.5, -437.5) -> (0, -437.5)
  line L166 (0, -437.5) -> (0, -446.5)
  line L167 (0, -446.5) -> (17.5, -446.5)
  line L168 (17.5, -446.5) -> (17.5, -447.5)
  line L169 (17.5, -447.5) -> (0, -447.5)
  line L170 (0, -447.5) -> (0, -456.5)
  line L171 (0, -456.5) -> (17.5, -456.5)
  line L172 (17.5, -456.5) -> (17.5, -457.5)
  line L173 (17.5, -457.5) -> (0, -457.5)
  line L174 (0, -457.5) -> (0, -466.5)
  line L175 (0, -466.5) -> (17.5, -466.5)
  line L176 (17.5, -466.5) -> (17.5, -467.5)
  line L177 (17.5, -467.5) -> (0, -467.5)
  line L178 (0, -467.5) -> (0, -476.5)
  line L179 (0, -476.5) -> (17.5, -476.5)
  line L180 (17.5, -476.5) -> (17.5, -477.5)
  line L181 (17.5, -477.5) -> (0, -477.5)
  line L182 (0, -477.5) -> (0, -486.5)
  line L183 (0, -486.5) -> (17.5, -486.5)
  line L184 (17.5, -486.5) -> (17.5, -487.5)
  line L185 (17.5, -487.5) -> (0, -487.5)
  line L186 (0, -487.5) -> (0, -496.5)
  line L187 (0, -496.5) -> (17.5, -496.5)
  line L188 (17.5, -496.5) -> (17.5, -497.5)
  line L189 (17.5, -497.5) -> (0, -497.5)
  line L190 (0, -497.5) -> (0, -506.5)
  line L191 (0, -506.5) -> (17.5, -506.5)
  line L192 (17.5, -506.5) -> (17.5, -507.5)
  line L193 (17.5, -507.5) -> (0, -507.5)
  line L194 (0, -507.5) -> (0, -516.5)
  line L195 (0, -516.5) -> (17.5, -516.5)
  line L196 (17.5, -516.5) -> (17.5, -517.5)
  line L197 (17.5, -517.5) -> (0, -517.5)
  line L198 (0, -517.5) -> (0, -526.5)
  line L199 (0, -526.5) -> (17.5, -526.5)
  line L200 (17.5, -526.5) -> (17.5, -527.5)
  line L201 (17.5, -527.5) -> (0, -527.5)
  line L202 (0, -527.5) -> (0, -536.5)
  line L203 (0, -536.5) -> (17.5, -536.5)
  line L204 (17.5, -536.5) -> (17.5, -537.5)
  line L205 (17.5, -537.5) -> (0, -537.5)
  line L206 (0, -537.5) -> (0, -546.5)
  line L207 (0, -546.5) -> (17.5, -546.5)
  line L208 (17.5, -546.5) -> (17.5, -547.5)
  line L209 (17.5, -547.5) -> (0, -547.5)
  line L210 (0, -547.5) -> (0, -556.5)
  line L211 (0, -556.5) -> (17.5, -556.5)
  line L212 (17.5, -556.5) -> (17.5, -557.5)
  line L213 (17.5, -557.5) -> (0, -557.5)
  line L214 (0, -557.5) -> (0, -566.5)
  line L215 (0, -566.5) -> (17.5, -566.5)
  line L216 (17.5, -566.5) -> (17.5, -567.5)
  line L217 (17.5, -567.5) -> (0, -567.5)
  line L218 (0, -567.5) -> (0, -576.5)
  line L219 (0, -576.5) -> (17.5, -576.5)
  line L220 (17.5, -576.5) -> (17.5, -577.5)
  line L221 (17.5, -577.5) -> (0, -577.5)
  line L222 (0, -577.5) -> (0, -586.5)
  line L223 (0, -586.5) -> (17.5, -586.5)
  line L224 (17.5, -586.5) -> (17.5, -587.5)
  line L225 (17.5, -587.5) -> (0, -587.5)
  line L226 (0, -587.5) -> (0, -596.5)
  line L227 (0, -596.5) -> (17.5, -596.5)
  line L228 (17.5, -596.5) -> (17.5, -597.5)
  line L229 (17.5, -597.5) -> (0, -597.5)
  line L230 (0, -597.5) -> (0, -606.5)
  line L231 (0, -606.5) -> (17.5, -606.5)
  line L232 (17.5, -606.5) -> (17.5, -607.5)
  line L233 (17.5, -607.5) -> (0, -607.5)
  line L234 (0, -607.5) -> (0, -616.5)
  line L235 (0, -616.5) -> (17.5, -616.5)
  line L236 (17.5, -616.5) -> (17.5, -617.5)
  line L237 (17.5, -617.5) -> (0, -617.5)
  line L238 (0, -617.5) -> (0, -626.5)
  line L239 (0, -626.5) -> (17.5, -626.5)
  line L240 (17.5, -626.5) -> (17.5, -627.5)
  line L241 (17.5, -627.5) -> (0, -627.5)
  line L242 (0, -627.5) -> (0, -636.5)
  line L243 (0, -636.5) -> (17.5, -636.5)
  line L244 (17.5, -636.5) -> (17.5, -637.5)
  line L245 (17.5, -637.5) -> (0, -637.5)
  line L246 (0, -637.5) -> (0, -646.5)
  line L247 (0, -646.5) -> (17.5, -646.5)
  line L248 (17.5, -646.5) -> (17.5, -647.5)
  line L249 (17.5, -647.5) -> (0, -647.5)
  line L250 (0, -647.5) -> (0, -656.5)
  line L251 (0, -656.5) -> (17.5, -656.5)
  line L252 (17.5, -656.5) -> (17.5, -657.5)
  line L253 (17.5, -657.5) -> (0, -657.5)
  line L254 (0, -657.5) -> (0, -666.5)
  line L255 (0, -666.5) -> (17.5, -666.5)
  line L256 (17.5, -666.5) -> (17.5, -667.5)
  line L257 (17.5, -667.5) -> (0, -667.5)
  line L258 (0, -667.5) -> (0, -676.5)
  line L259 (0, -676.5) -> (17.5, -676.5)
  line L260 (17.5, -676.5) -> (17.5, -677.5)
  line L261 (17.5, -677.5) -> (0, -677.5)
  line L262 (0, -677.5) -> (0, -686.5)
  line L263 (0, -686.5) -> (17.5, -686.5)
  line L264 (17.5, -686.5) -> (17.5, -687.5)
  line L265 (17.5, -687.5) -> (0, -687.5)
  line L266 (0, -687.5) -> (0, -696.5)
  line L267 (0, -696.5) -> (17.5, -696.5)
  line L268 (17.5, -696.5) -> (17.5, -697.5)
  line L269 (17.5, -697.5) -> (0, -697.5)
  line L270 (0, -697.5) -> (0, -706.5)
  line L271 (0, -706.5) -> (17.5, -706.5)
  line L272 (17.5, -706.5) -> (17.5, -707.5)
  line L273 (17.5, -707.5) -> (0, -707.5)
  line L274 (0, -707.5) -> (0, -716.5)
  line L275 (0, -716.5) -> (17.5, -716.5)
  line L276 (17.5, -716.5) -> (17.5, -717.5)
  line L277 (17.5, -717.5) -> (0, -717.5)
  line L278 (0, -717.5) -> (0, -726.5)
  line L279 (0, -726.5) -> (17.5, -726.5)
  line L280 (17.5, -726.5) -> (17.5, -727.5)
  line L281 (17.5, -727.5) -> (0, -727.5)
  line L282 (0, -727.5) -> (0, -736.5)
  line L283 (0, -736.5) -> (17.5, -736.5)
  line L284 (17.5, -736.5) -> (17.5, -737.5)
  line L285 (17.5, -737.5) -> (0, -737.5)
  line L286 (0, -737.5) -> (0, -746.5)
  line L287 (0, -746.5) -> (17.5, -746.5)
  line L288 (17.5, -746.5) -> (17.5, -747.5)
  line L289 (17.5, -747.5) -> (0, -747.5)
  line L290 (0, -747.5) -> (0, -756.5)
  line L291 (0, -756.5) -> (17.5, -756.5)
  line L292 (17.5, -756.5) -> (17.5, -757.5)
  line L293 (17.5, -757.5) -> (0, -757.5)
  line L294 (0, -757.5) -> (0, -766.5)
  line L295 (0, -766.5) -> (17.5, -766.5)
  line L296 (17.5, -766.5) -> (17.5, -767.5)
  line L297 (17.5, -767.5) -> (0, -767.5)
  line L298 (0, -767.5) -> (0, -776.5)
  line L299 (0, -776.5) -> (17.5, -776.5)
  line L300 (17.5, -776.5) -> (17.5, -777.5)
  line L301 (17.5, -777.5) -> (0, -777.5)
  line L302 (0, -777.5) -> (0, -786.5)
  line L303 (0, -786.5) -> (17.5, -786.5)
  line L304 (17.5, -786.5) -> (17.5, -787.5)
  line L305 (17.5, -787.5) -> (0, -787.5)
  line L306 (0, -787.5) -> (0, -796.5)
  line L307 (0, -796.5) -> (17.5, -796.5)
  line L308 (17.5, -796.5) -> (17.5, -797.5)
  line L309 (17.5, -797.5) -> (0, -797.5)
  line L310 (0, -797.5) -> (0, -806.5)
  line L311 (0, -806.5) -> (17.5, -806.5)
  line L312 (17.5, -806.5) -> (17.5, -807.5)
  line L313 (17.5, -807.5) -> (0, -807.5)
  line L314 (0, -807.5) -> (0, -816.5)
  line L315 (0, -816.5) -> (17.5, -816.5)
  line L316 (17.5, -816.5) -> (17.5, -817.5)
  line L317 (17.5, -817.5) -> (0, -817.5)
  line L318 (0, -817.5) -> (0, -826.5)
  line L319 (0, -826.5) -> (17.5, -826.5)
  line L320 (17.5, -826.5) -> (17.5, -827.5)
  line L321 (17.5, -827.5) -> (0, -827.5)
  line L322 (0, -827.5) -> (0, -836.5)
  line L323 (0, -836.5) -> (17.5, -836.5)
  line L324 (17.5, -836.5) -> (17.5, -837.5)
  line L325 (17.5, -837.5) -> (0, -837.5)
  line L326 (0, -837.5) -> (0, -870.7)
  line L327 (0, -870.7) -> (5, -870.7)
  line L328 (5, -870.7) -> (5, -884)
  line L329 (5, -884) -> (35, -884)
  line L330 (35, -884) -> (35, -870.7)
  line L331 (35, -870.7) -> (40, -870.7)
  line L332 (40, -870.7) -> (40, -3)
  line L333 (40, -3) -> (35, -3)
  line L334 (35, -3) -> (35, 10)
  line L335 (35, 10) -> (5, 10)
  line L336 (28.545, -839.4996) -> (28.5449, -835.8775)
  line L337 (28.5449, -835.8775) -> (29.094, -835.8775)
  line L338 (29.094, -835.8775) -> (29.094, -836.3857)
  spline S0 degree 3 poles (29.094, -836.3857) (29.1559, -836.3011) (29.2808, -836.1306) (29.4582, -836.0156) (29.5476, -835.9576) knots 0 0 0 0 0.031158 0.062835 0.062835 0.062835 0.062835
  spline S1 degree 3 poles (29.5476, -835.9576) (29.6468, -835.9104) (29.8507, -835.8133) (30.0763, -835.8016) (30.1922, -835.7956) knots 0 0 0 0 0.032617 0.067048 0.067048 0.067048 0.067048
  spline S2 degree 3 poles (30.1922, -835.7956) (30.3167, -835.8003) (30.5491, -835.8092) (30.7561, -835.914) (30.8522, -835.9627) knots 0 0 0 0 0.036859 0.068796 0.068796 0.068796 0.068796
  spline S3 degree 3 poles (30.8522, -835.9627) (30.9319, -836.0244) (31.0928, -836.1491) (31.1743, -836.3357) (31.2154, -836.4299) knots 0 0 0 0 0.029725 0.060035 0.060035 0.060035 0.060035
  spline S4 degree 3 poles (31.2154, -836.4299) (31.3656, -836.245) (31.6567, -835.8864) (32.1131, -835.8252) (32.3341, -835.7955) knots 0 0 0 0 0.068625 0.133024 0.133024 0.133024 0.133024
  spline S5 degree 3 poles (32.3341, -835.7955) (32.4992, -835.8039) (32.8071, -835.8196) (33.0502, -836.007) (33.1629, -836.0939) knots 0 0 0 0 0.048244 0.08997 0.08997 0.08997 0.08997
  spline S6 degree 3 poles (33.1629, -836.0939) (33.2472, -836.2162) (33.4366, -836.4911) (33.4471, -836.8268) (33.4528, -837.0131) knots 0 0 0 0 0.043695 0.098195 0.098195 0.098195 0.098195
  line L339 (33.4528, -837.0131) -> (33.4529, -839.4994)
  line L340 (33.4529, -839.4994) -> (32.8424, -839.4995)
  line L341 (32.8424, -839.4995) -> (32.8423, -837.2177)
  spline S7 degree 3 poles (32.8423, -837.2177) (32.8423, -837.1115) (32.8423, -836.9322) (32.7999, -836.7583) (32.7826, -836.6874) knots 0 0 0 0 0.031711 0.053535 0.053535 0.053535 0.053535
  spline S8 degree 3 poles (32.7826, -836.6874) (32.7582, -836.6357) (32.7084, -836.5303) (32.6141, -836.4615) (32.5661, -836.4265) knots 0 0 0 0 0.016863 0.034394 0.034394 0.034394 0.034394
  spline S9 degree 3 poles (32.5661, -836.4265) (32.5103, -836.3976) (32.3949, -836.3379) (32.2649, -836.3311) (32.1977, -836.3276) knots 0 0 0 0 0.018597 0.038532 0.038532 0.038532 0.038532
  spline S10 degree 3 poles (32.1977, -836.3276) (32.0766, -836.3374) (31.8386, -836.3566) (31.654, -836.5076) (31.5633, -836.5817) knots 0 0 0 0 0.035532 0.069798 0.069798 0.069798 0.069798
  spline S11 degree 3 poles (31.5633, -836.5817) (31.49, -836.6884) (31.3229, -836.9316) (31.3153, -837.2285) (31.311, -837.3951) knots 0 0 0 0 0.038079 0.086792 0.086792 0.086792 0.086792
  line L342 (31.311, -837.3951) -> (31.311, -839.4995)
  line L343 (31.311, -839.4995) -> (30.6971, -839.4995)
  line L344 (30.6971, -839.4995) -> (30.697, -837.1462)
  spline S12 degree 3 poles (30.697, -837.1462) (30.6946, -837.0241) (30.6903, -836.8074) (30.5906, -836.6159) (30.547, -836.5323) knots 0 0 0 0 0.036008 0.063954 0.063954 0.063954 0.063954
  spline S13 degree 3 poles (30.547, -836.5323) (30.4847, -836.4727) (30.3485, -836.3423) (30.1589, -836.3328) (30.0558, -836.3277) knots 0 0 0 0 0.025037 0.054812 0.054812 0.054812 0.054812
  spline S14 degree 3 poles (30.0558, -836.3277) (29.9711, -836.3333) (29.8016, -836.3447) (29.6516, -836.4243) (29.5766, -836.4641) knots 0 0 0 0 0.025172 0.050327 0.050327 0.050327 0.050327
  spline S15 degree 3 poles (29.5766, -836.4641) (29.508, -836.5158) (29.3677, -836.6214) (29.2949, -836.7814) (29.2577, -836.8631) knots 0 0 0 0 0.025339 0.051812 0.051812 0.051812 0.051812
  spline S16 degree 3 poles (29.2577, -836.8631) (29.229, -836.9694) (29.1622, -837.217) (29.1601, -837.4738) (29.1589, -837.6203) knots 0 0 0 0 0.032907 0.076633 0.076633 0.076633 0.076633
  line L345 (29.1589, -837.6203) -> (29.1589, -839.4996)
  line L346 (29.1589, -839.4996) -> (28.545, -839.4996)
  line L347 (19.0617, -788.1561) -> (19.7063, -788.1015)
  spline S17 degree 3 poles (19.7063, -788.1015) (19.734, -788.2447) (19.7853, -788.5096) (19.9591, -788.7149) (20.0389, -788.8091) knots 0 0 0 0 0.042908 0.079365 0.079365 0.079365 0.079365
  spline S18 degree 3 poles (20.0389, -788.8091) (20.1311, -788.8783) (20.3177, -789.0182) (20.5504, -789.0368) (20.6682, -789.0461) knots 0 0 0 0 0.033826 0.068485 0.068485 0.068485 0.068485
  spline S19 degree 3 poles (20.6682, -789.0461) (20.8106, -789.0318) (21.0974, -789.003) (21.311, -788.8093) (21.4185, -788.7118) knots 0 0 0 0 0.041772 0.0841 0.0841 0.0841 0.0841
  spline S20 degree 3 poles (21.4185, -788.7118) (21.508, -788.5868) (21.6971, -788.3223) (21.7156, -787.9967) (21.7254, -787.825) knots 0 0 0 0 0.045186 0.095569 0.095569 0.095569 0.095569
  spline S21 degree 3 poles (21.7254, -787.825) (21.7163, -787.6627) (21.6992, -787.3564) (21.5163, -787.1114) (21.4303, -786.9963) knots 0 0 0 0 0.047557 0.089725 0.089725 0.089725 0.089725
  spline S22 degree 3 poles (21.4303, -786.9963) (21.3218, -786.9078) (21.0972, -786.7246) (20.8075, -786.7036) (20.6578, -786.6928) knots 0 0 0 0 0.040971 0.08482 0.08482 0.08482 0.08482
  spline S23 degree 3 poles (20.6578, -786.6928) (20.5622, -786.6979) (20.3748, -786.708) (20.2053, -786.7883) (20.1223, -786.8275) knots 0 0 0 0 0.028423 0.055689 0.055689 0.055689 0.055689
  spline S24 degree 3 poles (20.1223, -786.8275) (20.0475, -786.8751) (19.9006, -786.9683) (19.7977, -787.1085) (19.7472, -787.1772) knots 0 0 0 0 0.026342 0.051681 0.051681 0.051681 0.051681
  line L348 (19.7472, -787.1772) -> (19.1708, -787.1022)
  line L349 (19.1708, -787.1022) -> (19.6549, -784.5339)
  line L350 (19.6549, -784.5339) -> (22.1413, -784.5337)
  line L351 (22.1413, -784.5337) -> (22.1413, -785.1204)
  line L352 (22.1413, -785.1204) -> (20.1461, -785.1205)
  line L353 (20.1461, -785.1205) -> (19.8767, -786.4643)
  spline S25 degree 3 poles (19.8767, -786.4643) (20.0262, -786.3728) (20.3171, -786.1948) (20.6565, -786.165) (20.8215, -786.1505) knots 0 0 0 0 0.051785 0.100763 0.100763 0.100763 0.100763
  spline S26 degree 3 poles (20.8215, -786.1505) (21.0307, -786.1688) (21.4463, -786.2053) (21.7672, -786.4717) (21.9265, -786.604) knots 0 0 0 0 0.061424 0.122014 0.122014 0.122014 0.122014
  spline S27 degree 3 poles (21.9265, -786.604) (22.0578, -786.7694) (22.3287, -787.1108) (22.3605, -787.5461) (22.3768, -787.7704) knots 0 0 0 0 0.061868 0.127641 0.127641 0.127641 0.127641
  spline S28 degree 3 poles (22.3768, -787.7704) (22.3616, -787.9874) (22.3318, -788.4132) (22.0967, -788.7691) (21.9813, -788.9437) knots 0 0 0 0 0.064036 0.125703 0.125703 0.125703 0.125703
  spline S29 degree 3 poles (21.9813, -788.9437) (21.8036, -789.1208) (21.4405, -789.4825) (20.9292, -789.5278) (20.6682, -789.5509) knots 0 0 0 0 0.072854 0.148822 0.148822 0.148822 0.148822
  spline S30 degree 3 poles (20.6682, -789.5509) (20.455, -789.5382) (20.0475, -789.5138) (19.7138, -789.2803) (19.5546, -789.169) knots 0 0 0 0 0.062678 0.119794 0.119794 0.119794 0.119794
  spline S31 degree 3 poles (19.5546, -789.169) (19.426, -789.0286) (19.1617, -788.7403) (19.0956, -788.3542) (19.0617, -788.1561) knots 0 0 0 0 0.055877 0.114795 0.114795 0.114795 0.114795
  line L354 (27.4212, -788.1384) -> (28.0249, -788.2168)
  spline S32 degree 3 poles (28.0249, -788.2168) (27.9822, -788.4107) (27.9005, -788.7824) (27.6421, -789.0608) (27.5185, -789.194) knots 0 0 0 0 0.058356 0.111856 0.111856 0.111856 0.111856
  spline S33 degree 3 poles (27.5185, -789.194) (27.3724, -789.2969) (27.0723, -789.5084) (26.7057, -789.5339) (26.5175, -789.5471) knots 0 0 0 0 0.052559 0.107965 0.107965 0.107965 0.107965
  spline S34 degree 3 poles (26.5175, -789.5471) (26.2844, -789.5296) (25.8328, -789.4957) (25.4886, -789.2028) (25.322, -789.0611) knots 0 0 0 0 0.068154 0.132052 0.132052 0.132052 0.132052
  spline S35 degree 3 poles (25.322, -789.0611) (25.1905, -788.8704) (24.9026, -788.453) (24.8815, -787.9442) (24.87, -787.6679) knots 0 0 0 0 0.068157 0.149141 0.149141 0.149141 0.149141
  spline S36 degree 3 poles (24.87, -787.6679) (24.8763, -787.4827) (24.8883, -787.1302) (25.0077, -786.7986) (25.0643, -786.6413) knots 0 0 0 0 0.055211 0.105055 0.105055 0.105055 0.105055
  spline S37 degree 3 poles (25.0643, -786.6413) (25.1365, -786.5044) (25.2787, -786.2348) (25.5316, -786.0649) (25.656, -785.9813) knots 0 0 0 0 0.04564 0.089884 0.089884 0.089884 0.089884
  spline S38 degree 3 poles (25.656, -785.9813) (25.792, -785.9171) (26.0658, -785.7878) (26.3683, -785.7701) (26.5206, -785.7612) knots 0 0 0 0 0.044643 0.089955 0.089955 0.089955 0.089955
  spline S39 degree 3 poles (26.5206, -785.7612) (26.7043, -785.7706) (27.0522, -785.7884) (27.3468, -785.9726) (27.4858, -786.0596) knots 0 0 0 0 0.054149 0.102527 0.102527 0.102527 0.102527
  spline S40 degree 3 poles (27.4858, -786.0596) (27.6003, -786.1731) (27.8394, -786.4101) (27.9232, -786.7368) (27.9668, -786.9071) knots 0 0 0 0 0.047449 0.099081 0.099081 0.099081 0.099081
  line L355 (27.9668, -786.9071) -> (27.3699, -786.9992)
  spline S41 degree 3 poles (27.3699, -786.9992) (27.3391, -786.8878) (27.2816, -786.6804) (27.1356, -786.523) (27.0681, -786.4501) knots 0 0 0 0 0.034086 0.063475 0.063475 0.063475 0.063475
  spline S42 degree 3 poles (27.0681, -786.4501) (26.9911, -786.3964) (26.8338, -786.2867) (26.6423, -786.273) (26.5445, -786.266) knots 0 0 0 0 0.027619 0.056426 0.056426 0.056426 0.056426
  spline S43 degree 3 poles (26.5445, -786.266) (26.3979, -786.2791) (26.1087, -786.3048) (25.8958, -786.5016) (25.7908, -786.5986) knots 0 0 0 0 0.04285 0.084486 0.084486 0.084486 0.084486
  spline S44 degree 3 poles (25.7908, -786.5986) (25.7066, -786.7382) (25.5128, -787.0597) (25.5052, -787.4372) (25.501, -787.6508) knots 0 0 0 0 0.048123 0.11083 0.11083 0.11083 0.11083